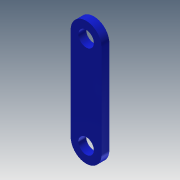
# Autodesk Inventor part: ruka_tahlo
Saved by Autodesk Inventor 2013 (Build 170138000, 138)
## iProperties
Created: 2013-02-01
Part Number: ruka_tahlo
Material: Generic
Document SubType Name: Modeling
Designer: idle-rug
Density: 1 g/cm^3
Author: idle-rug
Autodesk Inventor part; units mm, degrees
ref_plane "YZ Plane" through (0, 0, 0) normal (1, 0, 0) x (0, 1, 0)
ref_plane "XZ Plane" through (0, 0, 0) normal (0, 1, 0) x (-1, 0, 0)
ref_plane "XY Plane" through (0, 0, 0) normal (0, 0, 1) x (1, 0, 0)
sketch "Sketch1" plane through (0, 0, 0) normal (0, 1, 0) x (-1, 0, 0)
  line L0 (-3, -9) -> (3, -9)
  line L1 (3, -9) -> (3, 9)
  line L2 (3, 9) -> (-3, 9)
  line L3 (-3, 9) -> (-3, -9)
  line L4 (-3, -9) -> (3, 9) construction
  line L5 (3, -9) -> (-3, 9) construction
  circle A0 centre (0, -9) radius 3
  circle A1 centre (0, 9) radius 3
  point P0 (0, 0)
  dimension "d0" = 6
  dimension "d1" = 18
  dimension "d2" = 6
  constraints: 12 end point, 4 midpoint, 2 centre point, 2 parallel, 1 horizontal, 1 perpendicular, 1 tangent
  measures "d0" distance of L2.end L1.end
  measures "d1" distance of L1.end L0.end
  measures "d2" diameter of A1
extrude "Extrusion1" add sketch "Sketch1" along normal blind 1.5
sketch "Sketch2" plane through (0, 1.5, 0) normal (0, 1, 0) x (1, 0, 0)
  arc A0 (-3, -9) -> (3, -9) centre (0, -9) ccw projected
  arc A1 (3, 9) -> (-3, 9) centre (0, 9) ccw projected
  circle A2 centre (0, 9) radius 1.5
  circle A3 centre (0, -9) radius 1.5
  point P0 (0, 0)
  dimension "d5" = 3
  dimension "d6" = 3
  constraints: 2 centre point, 2 coincident
  measures "d5" diameter of A2
  measures "d6" diameter of A3
extrude "Extrusion2" cut sketch "Sketch2" against normal blind 2
body "Solid1"
